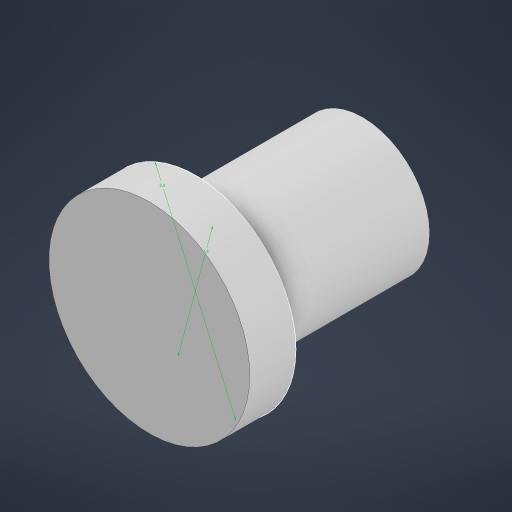
# Autodesk Inventor part: m1.6_4_なべ小ねじ0番
Saved by Autodesk Inventor 2023.5 (Build 275446000, 446)
## iProperties
Created: 2025-01-11
Part Number: m1.6_4_なべ小ねじ0番
Material: 一般
Document SubType Name: Modeling
Designer: IshiiLabHonda
Density: 1 g/cm^3
Appearance: 既定
Author: IshiiLabHonda
Autodesk Inventor part; units mm, degrees
ref_plane "YZ Plane" through (0, 0, 0) normal (1, 0, 0) x (0, 1, 0)
ref_plane "XZ Plane" through (0, 0, 0) normal (0, 1, 0) x (-1, 0, 0)
ref_plane "XY Plane" through (0, 0, 0) normal (0, 0, 1) x (1, 0, 0)
sketch "スケッチ2" plane through (0, 0, 0) normal (0, 0, 1) x (1, 0, 0)
  circle A0 centre (0, 0) radius 1.2
  circle A1 centre (0, 0) radius 0.8
  dimension "d1" = 2.4
  dimension "d2" = 1.6
  constraints: 2 centre point, 2 coincident
  measures "d1" diameter of A0
  measures "d2" diameter of A1
extrude "押し出し1" add sketch "スケッチ2" along normal blind 0.55 contours A0 | A1
extrude "押し出し2" add sketch "スケッチ2" against normal blind 2 contours A1
